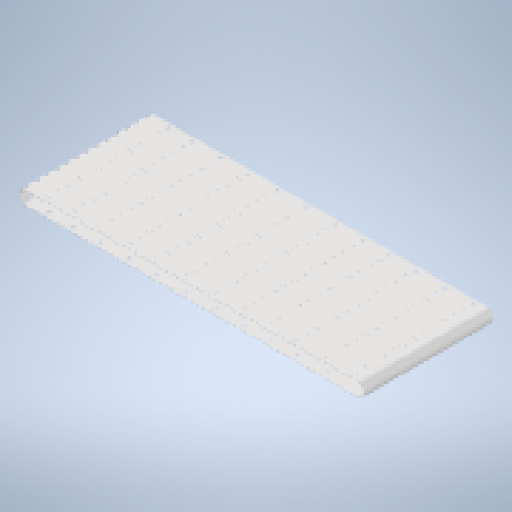
# Autodesk Inventor part: BangTai_Luoi_demo
Saved by Autodesk Inventor 2023 (Build 270158000, 158)
## iProperties
Created: 2025-04-18
Part Number: BangTai_Luoi_demo
Material: Generic
Document SubType Name: Modeling
Designer: huyqu
Density: 1 g/cm^3
Appearance: Default
Author: huyqu
Autodesk Inventor part; units mm, degrees
(part 1 of 2)
ref_plane "YZ Plane" through (0, 0, 0) normal (1, 0, 0) x (0, 1, 0)
ref_plane "XZ Plane" through (0, 0, 0) normal (0, 1, 0) x (-1, 0, 0)
ref_plane "XY Plane" through (0, 0, 0) normal (0, 0, 1) x (1, 0, 0)
sketch "Sketch1" plane through (0, 0, 0) normal (0, 0, 1) x (1, 0, 0)
  arc A0 (0.0295, 40) -> (-3.0425, -39.8841) centre (0, 0) ccw
  arc A1 (0.0295, 41.5) -> (-3.0425, -41.3883) centre (0, 0) ccw
  line L0 (0.0295, 41.5) -> (0.0295, 40)
  line L1 (-3.0425, -39.8841) -> (-3.0425, -41.3883)
  line L2 (0.0295, 41.5) -> (2000.0295, 41.5)
  line L3 (0.0295, 40) -> (2000.0295, 40)
  line L4 (-3.0425, -39.8841) -> (1996.9575, -39.8841)
  line L5 (-3.0425, -41.3883) -> (1996.9575, -41.3883)
  arc A2 (1996.9575, -39.8841) -> (2000.0295, 40) centre (2000, 0) ccw
  arc A3 (1996.9575, -41.3883) -> (2000.0295, 41.5) centre (2000, 0) ccw
  point P0 (-39.9705, 1.5371)
  dimension "d0" = 80
  dimension "d1" = 83
  dimension "d2" = 2000
  dimension "d3" = 2000
  dimension "d4" = 2000
  dimension "d5" = 2000
  dimension "d457" = 40
  constraints: 12 end point, 9 point on circle, 4 centre point, 4 horizontal, 3 coincident, 2 vertical
  measures "d0" diameter of A0
  measures "d1" diameter of A1
  measures "d2" distance of L2.end L0.start
  measures "d3" distance of L0.end L3.end
  measures "d4" distance of L1.start L4.end
  measures "d5" distance of L5.end L1.end
  measures "d457" distance from line of point (-39.97, 1.537) L0
extrude "Extrusion1" add sketch "Sketch1" along normal blind 780 contours A0 L1 A1 L0 | L0 L2 A3 L5 L1 L4 A2 L3
sketch "Sketch2" plane through (0.0295, 41.5, 0) normal (0, 1, 0) x (1, 0, 0)
  line L0 (-30, -20) -> (-10, -20)
  line L1 (-10, -20) -> (-10, -40)
  line L2 (-10, -40) -> (-30, -40)
  line L3 (-30, -40) -> (-30, -20)
  line L4 (0, 0) -> (0, -780) projected
  line L5 (-30, -80) -> (-10, -80)
  line L6 (-10, -80) -> (-10, -100)
  line L7 (-10, -100) -> (-30, -100)
  line L8 (-30, -100) -> (-30, -80)
  line L9 (-30, -140) -> (-10, -140)
  line L10 (-10, -140) -> (-10, -160)
  line L11 (-10, -160) -> (-30, -160)
  line L12 (-30, -160) -> (-30, -140)
  line L13 (-30, -200) -> (-10, -200)
  line L14 (-10, -200) -> (-10, -220)
  line L15 (-10, -220) -> (-30, -220)
  line L16 (-30, -220) -> (-30, -200)
  line L17 (-30, -380) -> (-10, -380)
  line L18 (-10, -380) -> (-10, -400)
  line L19 (-10, -400) -> (-30, -400)
  line L20 (-30, -400) -> (-30, -380)
  line L21 (-30, -440) -> (-10, -440)
  line L22 (-10, -440) -> (-10, -460)
  line L23 (-10, -460) -> (-30, -460)
  line L24 (-30, -460) -> (-30, -440)
  line L25 (-30, -500) -> (-10, -500)
  line L26 (-10, -500) -> (-10, -520)
  line L27 (-10, -520) -> (-30, -520)
  line L28 (-30, -520) -> (-30, -500)
  line L29 (-30, -560) -> (-10, -560)
  line L30 (-10, -560) -> (-10, -580)
  line L31 (-10, -580) -> (-30, -580)
  line L32 (-30, -580) -> (-30, -560)
  line L33 (-30, -620) -> (-10, -620)
  line L34 (-10, -620) -> (-10, -640)
  line L35 (-10, -640) -> (-30, -640)
  line L36 (-30, -640) -> (-30, -620)
  line L37 (-30, -680) -> (-10, -680)
  line L38 (-10, -680) -> (-10, -700)
  line L39 (-10, -700) -> (-30, -700)
  line L40 (-30, -700) -> (-30, -680)
  line L41 (-30, -740) -> (-10, -740)
  line L42 (-10, -740) -> (-10, -760)
  line L43 (-10, -760) -> (-30, -760)
  line L44 (-30, -760) -> (-30, -740)
  line L45 (-41.5295, 0) -> (-0.0295, 0) projected
  line L46 (-41.5295, -780) -> (0, -780) projected
  line L47 (-30, -260) -> (-10, -260)
  line L48 (-10, -260) -> (-10, -280)
  line L49 (-10, -280) -> (-30, -280)
  line L50 (-30, -280) -> (-30, -260)
  line L51 (-30, -320) -> (-10, -320)
  line L52 (-10, -320) -> (-10, -340)
  line L53 (-30, -340) -> (-30, -320)
  line L54 (-10, -340) -> (-30, -340)
  line L55 (99.353, -20) -> (119.353, -20)
  line L56 (119.353, -20) -> (119.353, -40)
  line L57 (119.353, -40) -> (99.353, -40)
  line L58 (99.353, -40) -> (99.353, -20)
  line L59 (99.353, -80) -> (119.353, -80)
  line L60 (119.353, -80) -> (119.353, -100)
  line L61 (119.353, -100) -> (99.353, -100)
  line L62 (99.353, -100) -> (99.353, -80)
  line L63 (99.353, -140) -> (119.353, -140)
  line L64 (119.353, -140) -> (119.353, -160)
  line L65 (119.353, -160) -> (99.353, -160)
  line L66 (99.353, -160) -> (99.353, -140)
  line L67 (99.353, -200) -> (119.353, -200)
  line L68 (119.353, -200) -> (119.353, -220)
  line L69 (119.353, -220) -> (99.353, -220)
  line L70 (99.353, -220) -> (99.353, -200)
  line L71 (99.353, -380) -> (119.353, -380)
  line L72 (119.353, -380) -> (119.353, -400)
  line L73 (119.353, -400) -> (99.353, -400)
  line L74 (99.353, -400) -> (99.353, -380)
  line L75 (99.353, -440) -> (119.353, -440)
  line L76 (119.353, -440) -> (119.353, -460)
  line L77 (119.353, -460) -> (99.353, -460)
  line L78 (99.353, -460) -> (99.353, -440)
  line L79 (99.353, -500) -> (119.353, -500)
  line L80 (119.353, -500) -> (119.353, -520)
  line L81 (119.353, -520) -> (99.353, -520)
  line L82 (99.353, -520) -> (99.353, -500)
  line L83 (99.353, -560) -> (119.353, -560)
  line L84 (119.353, -560) -> (119.353, -580)
  line L85 (119.353, -580) -> (99.353, -580)
  line L86 (99.353, -580) -> (99.353, -560)
  line L87 (99.353, -620) -> (119.353, -620)
  line L88 (119.353, -620) -> (119.353, -640)
  line L89 (119.353, -640) -> (99.353, -640)
  line L90 (99.353, -640) -> (99.353, -620)
  line L91 (99.353, -680) -> (119.353, -680)
  line L92 (119.353, -680) -> (119.353, -700)
  line L93 (119.353, -700) -> (99.353, -700)
  line L94 (99.353, -700) -> (99.353, -680)
  line L95 (99.353, -740) -> (119.353, -740)
  line L96 (119.353, -740) -> (119.353, -760)
  line L97 (119.353, -760) -> (99.353, -760)
  line L98 (99.353, -760) -> (99.353, -740)
  line L99 (99.353, -260) -> (119.353, -260)
  line L100 (119.353, -260) -> (119.353, -280)
  line L101 (99.353, -280) -> (99.353, -260)
  line L102 (119.353, -280) -> (99.353, -280)
  line L103 (99.353, -320) -> (119.353, -320)
  line L104 (119.353, -320) -> (119.353, -340)
  line L105 (99.353, -340) -> (99.353, -320)
  line L106 (119.353, -340) -> (99.353, -340)
  line L107 (245.8964, -20) -> (265.8964, -20)
  line L108 (265.8964, -20) -> (265.8964, -40)
  line L109 (265.8964, -40) -> (245.8964, -40)
  line L110 (245.8964, -40) -> (245.8964, -20)
  line L111 (245.8964, -80) -> (265.8964, -80)
  line L112 (265.8964, -80) -> (265.8964, -100)
  line L113 (265.8964, -100) -> (245.8964, -100)
  line L114 (245.8964, -100) -> (245.8964, -80)
  line L115 (245.8964, -140) -> (265.8964, -140)
  line L116 (265.8964, -140) -> (265.8964, -160)
  line L117 (265.8964, -160) -> (245.8964, -160)
  line L118 (245.8964, -160) -> (245.8964, -140)
  line L119 (245.8964, -200) -> (265.8964, -200)
  line L120 (265.8964, -200) -> (265.8964, -220)
  line L121 (265.8964, -220) -> (245.8964, -220)
  line L122 (245.8964, -220) -> (245.8964, -200)
  line L123 (245.8964, -380) -> (265.8964, -380)
  line L124 (265.8964, -380) -> (265.8964, -400)
  line L125 (265.8964, -400) -> (245.8964, -400)
  line L126 (245.8964, -400) -> (245.8964, -380)
  line L127 (245.8964, -440) -> (265.8964, -440)
  line L128 (265.8964, -440) -> (265.8964, -460)
  line L129 (265.8964, -460) -> (245.8964, -460)
  line L130 (245.8964, -460) -> (245.8964, -440)
  line L131 (245.8964, -500) -> (265.8964, -500)
  line L132 (265.8964, -500) -> (265.8964, -520)
  line L133 (265.8964, -520) -> (245.8964, -520)
  line L134 (245.8964, -520) -> (245.8964, -500)
  line L135 (245.8964, -560) -> (265.8964, -560)
  line L136 (265.8964, -560) -> (265.8964, -580)
  line L137 (265.8964, -580) -> (245.8964, -580)
  line L138 (245.8964, -580) -> (245.8964, -560)
  line L139 (245.8964, -620) -> (265.8964, -620)
  line L140 (265.8964, -620) -> (265.8964, -640)
  line L141 (265.8964, -640) -> (245.8964, -640)
  line L142 (245.8964, -640) -> (245.8964, -620)
  line L143 (245.8964, -680) -> (265.8964, -680)
  line L144 (265.8964, -680) -> (265.8964, -700)
  line L145 (265.8964, -700) -> (245.8964, -700)
  line L146 (245.8964, -700) -> (245.8964, -680)
  line L147 (245.8964, -740) -> (265.8964, -740)
  line L148 (265.8964, -740) -> (265.8964, -760)
  line L149 (265.8964, -760) -> (245.8964, -760)
  line L150 (245.8964, -760) -> (245.8964, -740)
  line L151 (245.8964, -260) -> (265.8964, -260)
  line L152 (265.8964, -260) -> (265.8964, -280)
  line L153 (245.8964, -280) -> (245.8964, -260)
  line L154 (265.8964, -280) -> (245.8964, -280)
  line L155 (245.8964, -320) -> (265.8964, -320)
  line L156 (265.8964, -320) -> (265.8964, -340)
  line L157 (245.8964, -340) -> (245.8964, -320)
  line L158 (265.8964, -340) -> (245.8964, -340)
  line L159 (413.9508, -20) -> (433.9508, -20)
  line L160 (433.9508, -20) -> (433.9508, -40)
  line L161 (433.9508, -40) -> (413.9508, -40)
  line L162 (413.9508, -40) -> (413.9508, -20)
  line L163 (413.9508, -80) -> (433.9508, -80)
  line L164 (433.9508, -80) -> (433.9508, -100)
  line L165 (433.9508, -100) -> (413.9508, -100)
  line L166 (413.9508, -100) -> (413.9508, -80)
  line L167 (413.9508, -140) -> (433.9508, -140)
  line L168 (433.9508, -140) -> (433.9508, -160)
  line L169 (433.9508, -160) -> (413.9508, -160)
  line L170 (413.9508, -160) -> (413.9508, -140)
  line L171 (413.9508, -200) -> (433.9508, -200)
  line L172 (433.9508, -200) -> (433.9508, -220)
  line L173 (433.9508, -220) -> (413.9508, -220)
  line L174 (413.9508, -220) -> (413.9508, -200)
  line L175 (413.9508, -380) -> (433.9508, -380)
  line L176 (433.9508, -380) -> (433.9508, -400)
  line L177 (433.9508, -400) -> (413.9508, -400)
  line L178 (413.9508, -400) -> (413.9508, -380)
  line L179 (413.9508, -440) -> (433.9508, -440)
  line L180 (433.9508, -440) -> (433.9508, -460)
  line L181 (433.9508, -460) -> (413.9508, -460)
  line L182 (413.9508, -460) -> (413.9508, -440)
  line L183 (413.9508, -500) -> (433.9508, -500)
  line L184 (433.9508, -500) -> (433.9508, -520)
  line L185 (433.9508, -520) -> (413.9508, -520)
  line L186 (413.9508, -520) -> (413.9508, -500)
  line L187 (413.9508, -560) -> (433.9508, -560)
  line L188 (433.9508, -560) -> (433.9508, -580)
  line L189 (433.9508, -580) -> (413.9508, -580)
  line L190 (413.9508, -580) -> (413.9508, -560)
  line L191 (413.9508, -620) -> (433.9508, -620)
  line L192 (433.9508, -620) -> (433.9508, -640)
  line L193 (433.9508, -640) -> (413.9508, -640)
  line L194 (413.9508, -640) -> (413.9508, -620)
  line L195 (413.9508, -680) -> (433.9508, -680)
  line L196 (433.9508, -680) -> (433.9508, -700)
  line L197 (433.9508, -700) -> (413.9508, -700)
  line L198 (413.9508, -700) -> (413.9508, -680)
  line L199 (413.9508, -740) -> (433.9508, -740)
  line L200 (433.9508, -740) -> (433.9508, -760)
  line L201 (433.9508, -760) -> (413.9508, -760)
  line L202 (413.9508, -760) -> (413.9508, -740)
  line L203 (413.9508, -260) -> (433.9508, -260)
  line L204 (433.9508, -260) -> (433.9508, -280)
  line L205 (413.9508, -280) -> (413.9508, -260)
  line L206 (433.9508, -280) -> (413.9508, -280)
  line L207 (413.9508, -320) -> (433.9508, -320)
  line L208 (433.9508, -320) -> (433.9508, -340)
  line L209 (413.9508, -340) -> (413.9508, -320)
  line L210 (433.9508, -340) -> (413.9508, -340)
  line L211 (582.0051, -20) -> (602.0051, -20)
  line L212 (602.0051, -20) -> (602.0051, -40)
  line L213 (602.0051, -40) -> (582.0051, -40)
  line L214 (582.0051, -40) -> (582.0051, -20)
  line L215 (582.0051, -80) -> (602.0051, -80)
  line L216 (602.0051, -80) -> (602.0051, -100)
  line L217 (602.0051, -100) -> (582.0051, -100)
  line L218 (582.0051, -100) -> (582.0051, -80)
  line L219 (582.0051, -140) -> (602.0051, -140)
  line L220 (602.0051, -140) -> (602.0051, -160)
  line L221 (602.0051, -160) -> (582.0051, -160)
  line L222 (582.0051, -160) -> (582.0051, -140)
  line L223 (582.0051, -200) -> (602.0051, -200)
  line L224 (602.0051, -200) -> (602.0051, -220)
  line L225 (602.0051, -220) -> (582.0051, -220)
  line L226 (582.0051, -220) -> (582.0051, -200)
  line L227 (582.0051, -380) -> (602.0051, -380)
  line L228 (602.0051, -380) -> (602.0051, -400)
  line L229 (602.0051, -400) -> (582.0051, -400)
  line L230 (582.0051, -400) -> (582.0051, -380)
  line L231 (582.0051, -440) -> (602.0051, -440)
  line L232 (602.0051, -440) -> (602.0051, -460)
  line L233 (602.0051, -460) -> (582.0051, -460)
  line L234 (582.0051, -460) -> (582.0051, -440)
  line L235 (582.0051, -500) -> (602.0051, -500)
  line L236 (602.0051, -500) -> (602.0051, -520)
  line L237 (602.0051, -520) -> (582.0051, -520)
  line L238 (582.0051, -520) -> (582.0051, -500)
  line L239 (582.0051, -560) -> (602.0051, -560)
  line L240 (602.0051, -560) -> (602.0051, -580)
  line L241 (602.0051, -580) -> (582.0051, -580)
  line L242 (582.0051, -580) -> (582.0051, -560)
  line L243 (582.0051, -620) -> (602.0051, -620)
  line L244 (602.0051, -620) -> (602.0051, -640)
  line L245 (602.0051, -640) -> (582.0051, -640)
  line L246 (582.0051, -640) -> (582.0051, -620)
  line L247 (582.0051, -680) -> (602.0051, -680)
  line L248 (602.0051, -680) -> (602.0051, -700)
  line L249 (602.0051, -700) -> (582.0051, -700)
  line L250 (582.0051, -700) -> (582.0051, -680)
  line L251 (582.0051, -740) -> (602.0051, -740)
  line L252 (602.0051, -740) -> (602.0051, -760)
  line L253 (602.0051, -760) -> (582.0051, -760)
  line L254 (582.0051, -760) -> (582.0051, -740)
  line L255 (582.0051, -260) -> (602.0051, -260)
  line L256 (602.0051, -260) -> (602.0051, -280)
  line L257 (582.0051, -280) -> (582.0051, -260)
  line L258 (602.0051, -280) -> (582.0051, -280)
  line L259 (582.0051, -320) -> (602.0051, -320)
  line L260 (602.0051, -320) -> (602.0051, -340)
  line L261 (582.0051, -340) -> (582.0051, -320)
  line L262 (602.0051, -340) -> (582.0051, -340)
  line L263 (751.4039, -20) -> (771.4039, -20)
  line L264 (771.4039, -20) -> (771.4039, -40)
  line L265 (771.4039, -40) -> (751.4039, -40)
  line L266 (751.4039, -40) -> (751.4039, -20)
  line L267 (751.4039, -80) -> (771.4039, -80)
  line L268 (771.4039, -80) -> (771.4039, -100)
  line L269 (771.4039, -100) -> (751.4039, -100)
  line L270 (751.4039, -100) -> (751.4039, -80)
  line L271 (751.4039, -140) -> (771.4039, -140)
  line L272 (771.4039, -140) -> (771.4039, -160)
  line L273 (771.4039, -160) -> (751.4039, -160)
  line L274 (751.4039, -160) -> (751.4039, -140)
  line L275 (751.4039, -200) -> (771.4039, -200)
  line L276 (771.4039, -200) -> (771.4039, -220)
  line L277 (771.4039, -220) -> (751.4039, -220)
  line L278 (751.4039, -220) -> (751.4039, -200)
  line L279 (751.4039, -380) -> (771.4039, -380)
  line L280 (771.4039, -380) -> (771.4039, -400)
  line L281 (771.4039, -400) -> (751.4039, -400)
  line L282 (751.4039, -400) -> (751.4039, -380)
  line L283 (751.4039, -440) -> (771.4039, -440)
  line L284 (771.4039, -440) -> (771.4039, -460)
  line L285 (771.4039, -460) -> (751.4039, -460)
  line L286 (751.4039, -460) -> (751.4039, -440)
  line L287 (751.4039, -500) -> (771.4039, -500)
  line L288 (771.4039, -500) -> (771.4039, -520)
  line L289 (771.4039, -520) -> (751.4039, -520)
  line L290 (751.4039, -520) -> (751.4039, -500)
  line L291 (751.4039, -560) -> (771.4039, -560)
  line L292 (771.4039, -560) -> (771.4039, -580)
  line L293 (771.4039, -580) -> (751.4039, -580)
  line L294 (751.4039, -580) -> (751.4039, -560)
  line L295 (751.4039, -620) -> (771.4039, -620)
  line L296 (771.4039, -620) -> (771.4039, -640)
  line L297 (771.4039, -640) -> (751.4039, -640)
  line L298 (751.4039, -640) -> (751.4039, -620)
  line L299 (751.4039, -680) -> (771.4039, -680)
  line L300 (771.4039, -680) -> (771.4039, -700)
  line L301 (771.4039, -700) -> (751.4039, -700)
  line L302 (751.4039, -700) -> (751.4039, -680)
  line L303 (751.4039, -740) -> (771.4039, -740)
  line L304 (771.4039, -740) -> (771.4039, -760)
  line L305 (771.4039, -760) -> (751.4039, -760)
  line L306 (751.4039, -760) -> (751.4039, -740)
  line L307 (751.4039, -260) -> (771.4039, -260)
  line L308 (771.4039, -260) -> (771.4039, -280)
  line L309 (751.4039, -280) -> (751.4039, -260)
  line L310 (771.4039, -280) -> (751.4039, -280)
  line L311 (751.4039, -320) -> (771.4039, -320)
  line L312 (771.4039, -320) -> (771.4039, -340)
  line L313 (751.4039, -340) -> (751.4039, -320)
  line L314 (771.4039, -340) -> (751.4039, -340)
  line L315 (930.2137, -20) -> (950.2137, -20)
  line L316 (950.2137, -20) -> (950.2137, -40)
  line L317 (950.2137, -40) -> (930.2137, -40)
  line L318 (930.2137, -40) -> (930.2137, -20)
  line L319 (930.2137, -80) -> (950.2137, -80)
  line L320 (950.2137, -80) -> (950.2137, -100)
  line L321 (950.2137, -100) -> (930.2137, -100)
  line L322 (930.2137, -100) -> (930.2137, -80)
  line L323 (930.2137, -140) -> (950.2137, -140)
  line L324 (950.2137, -140) -> (950.2137, -160)
  line L325 (950.2137, -160) -> (930.2137, -160)
  line L326 (930.2137, -160) -> (930.2137, -140)
  line L327 (930.2137, -200) -> (950.2137, -200)
  line L328 (950.2137, -200) -> (950.2137, -220)
  line L329 (950.2137, -220) -> (930.2137, -220)
  line L330 (930.2137, -220) -> (930.2137, -200)
  line L331 (930.2137, -380) -> (950.2137, -380)
  line L332 (950.2137, -380) -> (950.2137, -400)
  line L333 (950.2137, -400) -> (930.2137, -400)
  line L334 (930.2137, -400) -> (930.2137, -380)
  line L335 (930.2137, -440) -> (950.2137, -440)
  line L336 (950.2137, -440) -> (950.2137, -460)
  line L337 (950.2137, -460) -> (930.2137, -460)
  line L338 (930.2137, -460) -> (930.2137, -440)
  line L339 (930.2137, -500) -> (950.2137, -500)
  line L340 (950.2137, -500) -> (950.2137, -520)
  line L341 (950.2137, -520) -> (930.2137, -520)
  line L342 (930.2137, -520) -> (930.2137, -500)
  line L343 (930.2137, -560) -> (950.2137, -560)
  line L344 (950.2137, -560) -> (950.2137, -580)
  line L345 (950.2137, -580) -> (930.2137, -580)
  line L346 (930.2137, -580) -> (930.2137, -560)
  line L347 (930.2137, -620) -> (950.2137, -620)
  line L348 (950.2137, -620) -> (950.2137, -640)
  line L349 (950.2137, -640) -> (930.2137, -640)
  line L350 (930.2137, -640) -> (930.2137, -620)
  line L351 (930.2137, -680) -> (950.2137, -680)
  line L352 (950.2137, -680) -> (950.2137, -700)
  line L353 (950.2137, -700) -> (930.2137, -700)
  line L354 (930.2137, -700) -> (930.2137, -680)
  line L355 (930.2137, -740) -> (950.2137, -740)
  line L356 (950.2137, -740) -> (950.2137, -760)
  line L357 (950.2137, -760) -> (930.2137, -760)
  line L358 (930.2137, -760) -> (930.2137, -740)
  line L359 (930.2137, -260) -> (950.2137, -260)
  line L360 (950.2137, -260) -> (950.2137, -280)
  line L361 (930.2137, -280) -> (930.2137, -260)
  line L362 (950.2137, -280) -> (930.2137, -280)
  line L363 (930.2137, -320) -> (950.2137, -320)
  line L364 (950.2137, -320) -> (950.2137, -340)
  line L365 (930.2137, -340) -> (930.2137, -320)
  line L366 (950.2137, -340) -> (930.2137, -340)
  line L367 (1109.0235, -20) -> (1129.0235, -20)
  line L368 (1129.0235, -20) -> (1129.0235, -40)
  line L369 (1129.0235, -40) -> (1109.0235, -40)
  line L370 (1109.0235, -40) -> (1109.0235, -20)
  line L371 (1109.0235, -80) -> (1129.0235, -80)
  line L372 (1129.0235, -80) -> (1129.0235, -100)
  line L373 (1129.0235, -100) -> (1109.0235, -100)
  line L374 (1109.0235, -100) -> (1109.0235, -80)
  line L375 (1109.0235, -140) -> (1129.0235, -140)
  line L376 (1129.0235, -140) -> (1129.0235, -160)
  line L377 (1129.0235, -160) -> (1109.0235, -160)
  line L378 (1109.0235, -160) -> (1109.0235, -140)
  line L379 (1109.0235, -200) -> (1129.0235, -200)
  line L380 (1129.0235, -200) -> (1129.0235, -220)
  line L381 (1129.0235, -220) -> (1109.0235, -220)
  line L382 (1109.0235, -220) -> (1109.0235, -200)
  line L383 (1109.0235, -380) -> (1129.0235, -380)
  line L384 (1129.0235, -380) -> (1129.0235, -400)
  line L385 (1129.0235, -400) -> (1109.0235, -400)
  line L386 (1109.0235, -400) -> (1109.0235, -380)
  line L387 (1109.0235, -440) -> (1129.0235, -440)
  line L388 (1129.0235, -440) -> (1129.0235, -460)
  line L389 (1129.0235, -460) -> (1109.0235, -460)
  line L390 (1109.0235, -460) -> (1109.0235, -440)
  line L391 (1109.0235, -500) -> (1129.0235, -500)
  line L392 (1129.0235, -500) -> (1129.0235, -520)
  line L393 (1129.0235, -520) -> (1109.0235, -520)
  line L394 (1109.0235, -520) -> (1109.0235, -500)
  line L395 (1109.0235, -560) -> (1129.0235, -560)
  line L396 (1129.0235, -560) -> (1129.0235, -580)
  line L397 (1129.0235, -580) -> (1109.0235, -580)
  line L398 (1109.0235, -580) -> (1109.0235, -560)
  line L399 (1109.0235, -620) -> (1129.0235, -620)
  line L400 (1129.0235, -620) -> (1129.0235, -640)
  line L401 (1129.0235, -640) -> (1109.0235, -640)
  line L402 (1109.0235, -640) -> (1109.0235, -620)
  line L403 (1109.0235, -680) -> (1129.0235, -680)
  line L404 (1129.0235, -680) -> (1129.0235, -700)
  line L405 (1129.0235, -700) -> (1109.0235, -700)
  line L406 (1109.0235, -700) -> (1109.0235, -680)
  line L407 (1109.0235, -740) -> (1129.0235, -740)
  line L408 (1129.0235, -740) -> (1129.0235, -760)
  line L409 (1129.0235, -760) -> (1109.0235, -760)
  line L410 (1109.0235, -760) -> (1109.0235, -740)
  line L411 (1109.0235, -260) -> (1129.0235, -260)
  line L412 (1129.0235, -260) -> (1129.0235, -280)
  line L413 (1109.0235, -280) -> (1109.0235, -260)
  line L414 (1129.0235, -280) -> (1109.0235, -280)
  line L415 (1109.0235, -320) -> (1129.0235, -320)
  line L416 (1129.0235, -320) -> (1129.0235, -340)
  line L417 (1109.0235, -340) -> (1109.0235, -320)
  line L418 (1129.0235, -340) -> (1109.0235, -340)
  line L419 (1276.7747, -20) -> (1296.7747, -20)
  line L420 (1296.7747, -20) -> (1296.7747, -40)
  line L421 (1296.7747, -40) -> (1276.7747, -40)
  line L422 (1276.7747, -40) -> (1276.7747, -20)
  line L423 (1276.7747, -80) -> (1296.7747, -80)
  line L424 (1296.7747, -80) -> (1296.7747, -100)
  line L425 (1296.7747, -100) -> (1276.7747, -100)
  line L426 (1276.7747, -100) -> (1276.7747, -80)
  line L427 (1276.7747, -140) -> (1296.7747, -140)
  line L428 (1296.7747, -140) -> (1296.7747, -160)
  line L429 (1296.7747, -160) -> (1276.7747, -160)
  line L430 (1276.7747, -160) -> (1276.7747, -140)
  line L431 (1276.7747, -200) -> (1296.7747, -200)
  line L432 (1296.7747, -200) -> (1296.7747, -220)
  line L433 (1296.7747, -220) -> (1276.7747, -220)
  line L434 (1276.7747, -220) -> (1276.7747, -200)
  line L435 (1276.7747, -380) -> (1296.7747, -380)
  line L436 (1296.7747, -380) -> (1296.7747, -400)
  line L437 (1296.7747, -400) -> (1276.7747, -400)
  line L438 (1276.7747, -400) -> (1276.7747, -380)
  line L439 (1276.7747, -440) -> (1296.7747, -440)
  line L440 (1296.7747, -440) -> (1296.7747, -460)
  line L441 (1296.7747, -460) -> (1276.7747, -460)
  line L442 (1276.7747, -460) -> (1276.7747, -440)
  line L443 (1276.7747, -500) -> (1296.7747, -500)
  line L444 (1296.7747, -500) -> (1296.7747, -520)
  line L445 (1296.7747, -520) -> (1276.7747, -520)
  line L446 (1276.7747, -520) -> (1276.7747, -500)
  line L447 (1276.7747, -560) -> (1296.7747, -560)
  line L448 (1296.7747, -560) -> (1296.7747, -580)
  line L449 (1296.7747, -580) -> (1276.7747, -580)
  line L450 (1276.7747, -580) -> (1276.7747, -560)
  line L451 (1276.7747, -620) -> (1296.7747, -620)
  line L452 (1296.7747, -620) -> (1296.7747, -640)
  line L453 (1296.7747, -640) -> (1276.7747, -640)
  line L454 (1276.7747, -640) -> (1276.7747, -620)
  line L455 (1276.7747, -680) -> (1296.7747, -680)
  line L456 (1296.7747, -680) -> (1296.7747, -700)
  line L457 (1296.7747, -700) -> (1276.7747, -700)
  line L458 (1276.7747, -700) -> (1276.7747, -680)
  line L459 (1276.7747, -740) -> (1296.7747, -740)
  line L460 (1296.7747, -740) -> (1296.7747, -760)
  line L461 (1296.7747, -760) -> (1276.7747, -760)
  line L462 (1276.7747, -760) -> (1276.7747, -740)
  line L463 (1276.7747, -260) -> (1296.7747, -260)
  line L464 (1296.7747, -260) -> (1296.7747, -280)
  line L465 (1276.7747, -280) -> (1276.7747, -260)
  line L466 (1296.7747, -280) -> (1276.7747, -280)
  line L467 (1276.7747, -320) -> (1296.7747, -320)
  line L468 (1296.7747, -320) -> (1296.7747, -340)
  line L469 (1276.7747, -340) -> (1276.7747, -320)
  line L470 (1296.7747, -340) -> (1276.7747, -340)
  line L471 (1429.1826, -20) -> (1449.1826, -20)
  line L472 (1449.1826, -20) -> (1449.1826, -40)
  line L473 (1449.1826, -40) -> (1429.1826, -40)
  line L474 (1429.1826, -40) -> (1429.1826, -20)
  line L475 (1429.1826, -80) -> (1449.1826, -80)
  line L476 (1449.1826, -80) -> (1449.1826, -100)
  line L477 (1449.1826, -100) -> (1429.1826, -100)
  line L478 (1429.1826, -100) -> (1429.1826, -80)
  line L479 (1429.1826, -140) -> (1449.1826, -140)
  line L480 (1449.1826, -140) -> (1449.1826, -160)
  line L481 (1449.1826, -160) -> (1429.1826, -160)
  line L482 (1429.1826, -160) -> (1429.1826, -140)
  line L483 (1429.1826, -200) -> (1449.1826, -200)
  line L484 (1449.1826, -200) -> (1449.1826, -220)
  line L485 (1449.1826, -220) -> (1429.1826, -220)
  line L486 (1429.1826, -220) -> (1429.1826, -200)
  line L487 (1429.1826, -380) -> (1449.1826, -380)
  line L488 (1449.1826, -380) -> (1449.1826, -400)
  line L489 (1449.1826, -400) -> (1429.1826, -400)
  line L490 (1429.1826, -400) -> (1429.1826, -380)
  line L491 (1429.1826, -440) -> (1449.1826, -440)
  line L492 (1449.1826, -440) -> (1449.1826, -460)
  line L493 (1449.1826, -460) -> (1429.1826, -460)
  line L494 (1429.1826, -460) -> (1429.1826, -440)
  line L495 (1429.1826, -500) -> (1449.1826, -500)
  line L496 (1449.1826, -500) -> (1449.1826, -520)
  line L497 (1449.1826, -520) -> (1429.1826, -520)
  line L498 (1429.1826, -520) -> (1429.1826, -500)
  line L499 (1429.1826, -560) -> (1449.1826, -560)
  line L500 (1449.1826, -560) -> (1449.1826, -580)
  line L501 (1449.1826, -580) -> (1429.1826, -580)
  line L502 (1429.1826, -580) -> (1429.1826, -560)
  line L503 (1429.1826, -620) -> (1449.1826, -620)
  line L504 (1449.1826, -620) -> (1449.1826, -640)
  line L505 (1449.1826, -640) -> (1429.1826, -640)
  line L506 (1429.1826, -640) -> (1429.1826, -620)
  line L507 (1429.1826, -680) -> (1449.1826, -680)
  line L508 (1449.1826, -680) -> (1449.1826, -700)
  line L509 (1449.1826, -700) -> (1429.1826, -700)
  line L510 (1429.1826, -700) -> (1429.1826, -680)
  line L511 (1429.1826, -740) -> (1449.1826, -740)
  line L512 (1449.1826, -740) -> (1449.1826, -760)
  line L513 (1449.1826, -760) -> (1429.1826, -760)
  line L514 (1429.1826, -760) -> (1429.1826, -740)
  line L515 (1429.1826, -260) -> (1449.1826, -260)
  line L516 (1449.1826, -260) -> (1449.1826, -280)
  line L517 (1429.1826, -280) -> (1429.1826, -260)
  line L518 (1449.1826, -280) -> (1429.1826, -280)
  line L519 (1429.1826, -320) -> (1449.1826, -320)
  line L520 (1449.1826, -320) -> (1449.1826, -340)
  line L521 (1429.1826, -340) -> (1429.1826, -320)
  line L522 (1449.1826, -340) -> (1429.1826, -340)
  line L523 (1592.0631, -20) -> (1612.0631, -20)
  line L524 (1612.0631, -20) -> (1612.0631, -40)
  line L525 (1612.0631, -40) -> (1592.0631, -40)
  line L526 (1592.0631, -40) -> (1592.0631, -20)
  line L527 (1592.0631, -80) -> (1612.0631, -80)
  line L528 (1612.0631, -80) -> (1612.0631, -100)
  line L529 (1612.0631, -100) -> (1592.0631, -100)
  line L530 (1592.0631, -100) -> (1592.0631, -80)
  line L531 (1592.0631, -140) -> (1612.0631, -140)
  line L532 (1612.0631, -140) -> (1612.0631, -160)
  line L533 (1612.0631, -160) -> (1592.0631, -160)
  line L534 (1592.0631, -160) -> (1592.0631, -140)
  line L535 (1592.0631, -200) -> (1612.0631, -200)
  line L536 (1612.0631, -200) -> (1612.0631, -220)
  line L537 (1612.0631, -220) -> (1592.0631, -220)
  line L538 (1592.0631, -220) -> (1592.0631, -200)
  line L539 (1592.0631, -380) -> (1612.0631, -380)
  line L540 (1612.0631, -380) -> (1612.0631, -400)
  line L541 (1612.0631, -400) -> (1592.0631, -400)
  line L542 (1592.0631, -400) -> (1592.0631, -380)
  line L543 (1592.0631, -440) -> (1612.0631, -440)
  line L544 (1612.0631, -440) -> (1612.0631, -460)
  line L545 (1612.0631, -460) -> (1592.0631, -460)
  line L546 (1592.0631, -460) -> (1592.0631, -440)
  line L547 (1592.0631, -500) -> (1612.0631, -500)
  line L548 (1612.0631, -500) -> (1612.0631, -520)
  line L549 (1612.0631, -520) -> (1592.0631, -520)
  line L550 (1592.0631, -520) -> (1592.0631, -500)
  line L551 (1592.0631, -560) -> (1612.0631, -560)
  line L552 (1612.0631, -560) -> (1612.0631, -580)
  line L553 (1612.0631, -580) -> (1592.0631, -580)
  line L554 (1592.0631, -580) -> (1592.0631, -560)
  line L555 (1592.0631, -620) -> (1612.0631, -620)
  line L556 (1612.0631, -620) -> (1612.0631, -640)
  line L557 (1612.0631, -640) -> (1592.0631, -640)
  line L558 (1592.0631, -640) -> (1592.0631, -620)
  line L559 (1592.0631, -680) -> (1612.0631, -680)
  line L560 (1612.0631, -680) -> (1612.0631, -700)
  line L561 (1612.0631, -700) -> (1592.0631, -700)
  line L562 (1592.0631, -700) -> (1592.0631, -680)
  line L563 (1592.0631, -740) -> (1612.0631, -740)
  line L564 (1612.0631, -740) -> (1612.0631, -760)
  line L565 (1612.0631, -760) -> (1592.0631, -760)
  line L566 (1592.0631, -760) -> (1592.0631, -740)
  line L567 (1592.0631, -260) -> (1612.0631, -260)
  line L568 (1612.0631, -260) -> (1612.0631, -280)
  line L569 (1592.0631, -280) -> (1592.0631, -260)
  line L570 (1612.0631, -280) -> (1592.0631, -280)
  line L571 (1592.0631, -320) -> (1612.0631, -320)
  line L572 (1612.0631, -320) -> (1612.0631, -340)
  line L573 (1592.0631, -340) -> (1592.0631, -320)
  line L574 (1612.0631, -340) -> (1592.0631, -340)
  line L575 (1770.5478, -20) -> (1790.5478, -20)
  line L576 (1790.5478, -20) -> (1790.5478, -40)
  line L577 (1790.5478, -40) -> (1770.5478, -40)
  line L578 (1770.5478, -40) -> (1770.5478, -20)
  line L579 (1770.5478, -80) -> (1790.5478, -80)
  line L580 (1790.5478, -80) -> (1790.5478, -100)
  line L581 (1790.5478, -100) -> (1770.5478, -100)
  line L582 (1770.5478, -100) -> (1770.5478, -80)
  line L583 (1770.5478, -140) -> (1790.5478, -140)
  line L584 (1790.5478, -140) -> (1790.5478, -160)
  line L585 (1790.5478, -160) -> (1770.5478, -160)
  line L586 (1770.5478, -160) -> (1770.5478, -140)
  line L587 (1770.5478, -200) -> (1790.5478, -200)
  line L588 (1790.5478, -200) -> (1790.5478, -220)
  line L589 (1790.5478, -220) -> (1770.5478, -220)
  line L590 (1770.5478, -220) -> (1770.5478, -200)
  line L591 (1770.5478, -380) -> (1790.5478, -380)
  line L592 (1790.5478, -380) -> (1790.5478, -400)
  line L593 (1790.5478, -400) -> (1770.5478, -400)
  line L594 (1770.5478, -400) -> (1770.5478, -380)
  line L595 (1770.5478, -440) -> (1790.5478, -440)
  line L596 (1790.5478, -440) -> (1790.5478, -460)
  line L597 (1790.5478, -460) -> (1770.5478, -460)
  line L598 (1770.5478, -460) -> (1770.5478, -440)
  line L599 (1770.5478, -500) -> (1790.5478, -500)
  line L600 (1790.5478, -500) -> (1790.5478, -520)
  line L601 (1790.5478, -520) -> (1770.5478, -520)
  line L602 (1770.5478, -520) -> (1770.5478, -500)
  line L603 (1770.5478, -560) -> (1790.5478, -560)
  line L604 (1790.5478, -560) -> (1790.5478, -580)
  line L605 (1790.5478, -580) -> (1770.5478, -580)
  line L606 (1770.5478, -580) -> (1770.5478, -560)
  line L607 (1770.5478, -620) -> (1790.5478, -620)
  line L608 (1790.5478, -620) -> (1790.5478, -640)
  line L609 (1790.5478, -640) -> (1770.5478, -640)
  line L610 (1770.5478, -640) -> (1770.5478, -620)
  line L611 (1770.5478, -680) -> (1790.5478, -680)
  line L612 (1790.5478, -680) -> (1790.5478, -700)
  line L613 (1790.5478, -700) -> (1770.5478, -700)
  line L614 (1770.5478, -700) -> (1770.5478, -680)
  line L615 (1770.5478, -740) -> (1790.5478, -740)
  line L616 (1790.5478, -740) -> (1790.5478, -760)
  line L617 (1790.5478, -760) -> (1770.5478, -760)
  line L618 (1770.5478, -760) -> (1770.5478, -740)
  line L619 (1770.5478, -260) -> (1790.5478, -260)
  line L620 (1790.5478, -260) -> (1790.5478, -280)
  line L621 (1770.5478, -280) -> (1770.5478, -260)
  line L622 (1790.5478, -280) -> (1770.5478, -280)
  line L623 (1770.5478, -320) -> (1790.5478, -320)
  line L624 (1790.5478, -320) -> (1790.5478, -340)
  line L625 (1770.5478, -340) -> (1770.5478, -320)
  line L626 (1790.5478, -340) -> (1770.5478, -340)
  point P0 (-20, -40)
  point P1 (-20, -100)
  point P2 (-20, -160)
  point P3 (-20, -220)
  point P4 (-20, -400)
  point P5 (-20, -460)
  point P6 (-20, -520)
  point P7 (-20, -580)
  point P8 (-20, -640)
  point P9 (-20, -700)
  point P10 (-20, -760)
  point P11 (-20, -740)
  point P12 (-20, -500)
  point P13 (-20, -280)
  point P14 (-20, -340)
  point P15 (109.353, -40)
  point P16 (109.353, -100)
  point P17 (109.353, -160)
  point P18 (109.353, -220)
  point P19 (109.353, -400)
  point P20 (109.353, -460)
  point P21 (109.353, -520)
  point P22 (109.353, -580)
  point P23 (109.353, -640)
  point P24 (109.353, -700)
  point P25 (109.353, -760)
  point P26 (109.353, -740)
  point P27 (109.353, -500)
  point P28 (109.353, -280)
  point P29 (109.353, -340)
  point P30 (255.8964, -40)
  point P31 (255.8964, -100)
  point P32 (255.8964, -160)
  point P33 (255.8964, -220)
  point P34 (255.8964, -400)
  point P35 (255.8964, -460)
  point P36 (255.8964, -520)
  point P37 (255.8964, -580)
  point P38 (255.8964, -640)
  point P39 (255.8964, -700)
  point P40 (255.8964, -760)
  point P41 (255.8964, -740)
  point P42 (255.8964, -500)
  point P43 (255.8964, -280)
  point P44 (255.8964, -340)
  point P45 (423.9508, -40)
  point P46 (423.9508, -100)
  point P47 (423.9508, -160)
  point P48 (423.9508, -220)
  point P49 (423.9508, -400)
  point P50 (423.9508, -460)
  point P51 (423.9508, -520)
  point P52 (423.9508, -580)
  point P53 (423.9508, -640)
  point P54 (423.9508, -700)
  point P55 (423.9508, -760)
  point P56 (423.9508, -740)
  point P57 (423.9508, -500)
  point P58 (423.9508, -280)
  point P59 (423.9508, -340)
  point P60 (592.0051, -40)
  point P61 (592.0051, -100)
  point P62 (592.0051, -160)
  point P63 (592.0051, -220)
  point P64 (592.0051, -400)
  point P65 (592.0051, -460)
  point P66 (592.0051, -520)
  point P67 (592.0051, -580)
  point P68 (592.0051, -640)
  point P69 (592.0051, -700)
  point P70 (592.0051, -760)
  point P71 (592.0051, -740)
  point P72 (592.0051, -500)
  point P73 (592.0051, -280)
  point P74 (592.0051, -340)
  point P75 (761.4039, -40)
  point P76 (761.4039, -100)
  point P77 (761.4039, -160)
  point P78 (761.4039, -220)
  point P79 (761.4039, -400)
  point P80 (761.4039, -460)
  point P81 (761.4039, -520)
  point P82 (761.4039, -580)
  point P83 (761.4039, -640)
  point P84 (761.4039, -700)
  point P85 (761.4039, -760)
  point P86 (761.4039, -740)
  point P87 (761.4039, -500)
  point P88 (761.4039, -280)
  point P89 (761.4039, -340)
  point P90 (940.2137, -40)
  point P91 (940.2137, -100)
  point P92 (940.2137, -160)
  point P93 (940.2137, -220)
  point P94 (940.2137, -400)
  point P95 (940.2137, -460)
  point P96 (940.2137, -520)
  point P97 (940.2137, -580)
  point P98 (940.2137, -640)
  point P99 (940.2137, -700)
  point P100 (940.2137, -760)
  point P101 (940.2137, -740)
  point P102 (940.2137, -500)
  point P103 (940.2137, -280)
  point P104 (940.2137, -340)
  point P105 (1119.0235, -40)
  point P106 (1119.0235, -100)
  point P107 (1119.0235, -160)
  point P108 (1119.0235, -220)
  point P109 (1119.0235, -400)
  point P110 (1119.0235, -460)
  point P111 (1119.0235, -520)
  point P112 (1119.0235, -580)
  point P113 (1119.0235, -640)
  point P114 (1119.0235, -700)
  point P115 (1119.0235, -760)
  point P116 (1119.0235, -740)
  point P117 (1119.0235, -500)
  point P118 (1119.0235, -280)
  point P119 (1119.0235, -340)
  point P120 (1286.7747, -40)
  point P121 (1286.7747, -100)
  point P122 (1286.7747, -160)
  point P123 (1286.7747, -220)
  point P124 (1286.7747, -400)
  point P125 (1286.7747, -460)
  point P126 (1286.7747, -520)
  point P127 (1286.7747, -580)
  point P128 (1286.7747, -640)
  point P129 (1286.7747, -700)
  point P130 (1286.7747, -760)
  point P131 (1286.7747, -740)
  point P132 (1286.7747, -500)
  point P133 (1286.7747, -280)
  point P134 (1286.7747, -340)
  point P135 (1439.1826, -40)
  point P136 (1439.1826, -100)
  point P137 (1439.1826, -160)
  point P138 (1439.1826, -220)
  point P139 (1439.1826, -400)
  point P140 (1439.1826, -460)
  point P141 (1439.1826, -520)
  point P142 (1439.1826, -580)
  point P143 (1439.1826, -640)
  point P144 (1439.1826, -700)
  point P145 (1439.1826, -760)
  point P146 (1439.1826, -740)
  point P147 (1439.1826, -500)
  point P148 (1439.1826, -280)
  point P149 (1439.1826, -340)
  point P150 (1602.0631, -40)
  point P151 (1602.0631, -100)
  point P152 (1602.0631, -160)
  point P153 (1602.0631, -220)
  point P154 (1602.0631, -400)
  point P155 (1602.0631, -460)
  point P156 (1602.0631, -520)
  point P157 (1602.0631, -580)
  point P158 (1602.0631, -640)
  point P159 (1602.0631, -700)
  point P160 (1602.0631, -760)
  point P161 (1602.0631, -740)
  point P162 (1602.0631, -500)
  point P163 (1602.0631, -280)
  point P164 (1602.0631, -340)
  point P165 (1780.5478, -40)
  point P166 (1780.5478, -100)
  point P167 (1780.5478, -160)
  point P168 (1780.5478, -220)
  point P169 (1780.5478, -400)
  point P170 (1780.5478, -460)
  point P171 (1780.5478, -520)
  point P172 (1780.5478, -580)
  point P173 (1780.5478, -640)
  point P174 (1780.5478, -700)
  point P175 (1780.5478, -760)
  point P176 (1780.5478, -740)
  point P177 (1780.5478, -500)
  point P178 (1780.5478, -280)
  point P179 (1780.5478, -340)
  dimension "d8" = 20
  dimension "d9" = 10
  dimension "d10" = 20
  dimension "d11" = 20
  dimension "d12" = 20
  dimension "d13" = 20
  dimension "d14" = 20
  dimension "d15" = 20
  dimension "d16" = 20
  dimension "d17" = 20
  dimension "d18" = 20
  dimension "d19" = 20
  dimension "d20" = 20
  dimension "d21" = 20
  dimension "d22" = 20
  dimension "d23" = 20
  dimension "d24" = 20
  dimension "d25" = 20
  dimension "d26" = 20
  dimension "d27" = 20
  dimension "d28" = 20
  dimension "d29" = 20
  dimension "d30" = 20
  dimension "d31" = 20
  dimension "d32" = 40
  dimension "d33" = 40
  dimension "d34" = 40
  dimension "d35" = 40
  dimension "d36" = 40
  dimension "d37" = 40
  dimension "d38" = 20
  dimension "d39" = 40
  dimension "d40" = 40
  dimension "d41" = 40
  dimension "d42" = 20
  dimension "d43" = 20
  dimension "d44" = 40
  dimension "d45" = 20
  dimension "d46" = 20
  dimension "d47" = 40
  dimension "d48" = 20
  dimension "d49" = 20
  dimension "d50" = 20
  dimension "d51" = 20
  dimension "d52" = 20
  dimension "d53" = 20
  dimension "d54" = 20
  dimension "d55" = 20
  dimension "d56" = 20
  dimension "d57" = 20
  dimension "d58" = 20
  dimension "d59" = 20
  dimension "d60" = 20
  dimension "d61" = 20
  dimension "d62" = 20
  dimension "d63" = 20
  dimension "d64" = 20
  dimension "d65" = 20
  dimension "d66" = 20
  dimension "d67" = 20
  dimension "d68" = 20
  dimension "d69" = 20
  dimension "d70" = 40
  dimension "d71" = 40
  constraints: 1248 end point, 312 parallel, 180 midpoint, 156 horizontal, 156 perpendicular
  measures "d8" distance from line of point (-20, -40) L0
  measures "d9" distance between parallel lines of L4 L1
  measures "d10" distance between parallel lines of L1 L3
  measures "d11" distance from line of point (-20, -100) L5
  measures "d12" distance between parallel lines of L6 L8
  measures "d13" distance from line of point (-20, -160) L9
  measures "d14" distance between parallel lines of L10 L12
  measures "d15" distance from line of point (-20, -220) L13
  measures "d16" distance between parallel lines of L14 L16
  measures "d17" distance from line of point (-20, -400) L17
  measures "d18" distance between parallel lines of L18 L20
  measures "d19" distance from line of point (-20, -460) L21
  measures "d20" distance between parallel lines of L22 L24
  measures "d21" distance from line of point (-20, -520) L25
  measures "d22" distance between parallel lines of L26 L28
  measures "d23" distance from line of point (-20, -580) L29
  measures "d24" distance between parallel lines of L30 L32
  measures "d25" distance from line of point (-20, -640) L33
  measures "d26" distance between parallel lines of L34 L36
  measures "d27" distance from line of point (-20, -700) L37
  measures "d28" distance between parallel lines of L38 L40
  measures "d29" distance from line of point (-20, -760) L41
  measures "d30" distance between parallel lines of L42 L44
  measures "d31" distance between parallel lines of L0 L45
  measures "d32" distance between parallel lines of L5 L2
  measures "d33" distance between parallel lines of L9 L7
  measures "d34" distance between parallel lines of L13 L11
  measures "d35" distance from line of point (-20, -740) L39
  measures "d36" distance between parallel lines of L37 L35
  measures "d37" distance between parallel lines of L33 L31
  measures "d38" distance between parallel lines of L46 L43
  measures "d39" distance between parallel lines of L29 L27
  measures "d40" distance from line of point (-20, -500) L23
  measures "d41" distance between parallel lines of L19 L21
  measures "d42" distance from line of point (-20, -280) L47
  measures "d43" distance between parallel lines of L48 L50
  measures "d44" distance between parallel lines of L47 L15
  measures "d45" distance from line of point (-20, -340) L51
  measures "d46" distance between parallel lines of L52 L53
  measures "d47" distance between parallel lines of L51 L49
  measures "d48" distance from line of point (109.353, -40) L55
  measures "d49" distance between parallel lines of L56 L58
  measures "d50" distance from line of point (109.353, -100) L59
  measures "d51" distance between parallel lines of L60 L62
  measures "d52" distance from line of point (109.353, -160) L63
  measures "d53" distance between parallel lines of L64 L66
  measures "d54" distance from line of point (109.353, -220) L67
  measures "d55" distance between parallel lines of L68 L70
  measures "d56" distance from line of point (109.353, -400) L71
  measures "d57" distance between parallel lines of L72 L74
  measures "d58" distance from line of point (109.353, -460) L75
  measures "d59" distance between parallel lines of L76 L78
  measures "d60" distance from line of point (109.353, -520) L79
  measures "d61" distance between parallel lines of L80 L82
  measures "d62" distance from line of point (109.353, -580) L83
  measures "d63" distance between parallel lines of L84 L86
  measures "d64" distance from line of point (109.353, -640) L87
  measures "d65" distance between parallel lines of L88 L90
  measures "d66" distance from line of point (109.353, -700) L91
  measures "d67" distance between parallel lines of L92 L94
  measures "d68" distance from line of point (109.353, -760) L95
  measures "d69" distance between parallel lines of L96 L98
  measures "d70" distance between parallel lines of L59 L57
  measures "d71" distance between parallel lines of L63 L61
extrude "Extrusion2" cut sketch "Sketch2" against normal through all